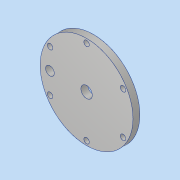
# Autodesk Inventor part: pistonSealingDisc
Saved by Autodesk Inventor 2017 (Build 210142000, 142)
## iProperties
Created: 2016-11-26
Part Number: pistonSealingDisc
Material: Aluminum 6061
Document SubType Name: Modeling
Designer: techn
Density: 2.7 g/cm^3
Appearance: Aluminum - Flat
Mass: 27.687 g
Surface Area: 74.4581 cm^2
Volume: 10.2545 cm^3
Author: techn
Autodesk Inventor part; units mm, degrees
ref_plane "YZ Plane" through (0, 0, 0) normal (1, 0, 0) x (0, 1, 0)
ref_plane "XZ Plane" through (0, 0, 0) normal (0, 1, 0) x (-1, 0, 0)
ref_plane "XY Plane" through (0, 0, 0) normal (0, 0, 1) x (1, 0, 0)
sketch "Sketch1" plane through (0, 0, 0) normal (0, 0, 1) x (1, 0, 0)
  circle A0 centre (0, 0) radius 32.1945
  dimension "d0" = 64.389
  constraints: 1 centre point, 1 coincident
  measures "d0" diameter of A0
extrude "Extrusion1" add sketch "Sketch1" along normal blind 4.7625
sketch "Sketch2" plane through (0, 0, 4.7625) normal (0, 0, 1) x (1, 0, 0)
  line L0 (0, 0) -> (0, 29.21)
  circle A0 centre (0, 29.21) radius 1.905
  circle A1 centre (-25.2966, 14.605) radius 1.905
  circle A2 centre (-25.2966, -14.605) radius 1.905
  circle A3 centre (0, -29.21) radius 1.905
  circle A4 centre (25.2966, -14.605) radius 1.905
  circle A5 centre (25.2966, 14.605) radius 1.905
  dimension "d3" = 29.21
  dimension "d4" = 3.81
  dimension "d7" = 360
  constraints: 6 centre point, 2 end point, 1 coincident, 1 vertical, 13 other
  measures "d3" distance of L0.start L0.end
  measures "d4" diameter of A0
extrude "Extrusion2" cut sketch "Sketch2" against normal through all
sketch "Sketch4" plane through (0, 0, 0) normal (0, 0, -1) x (-1, 0, 0)
  line L0 (0, 0) -> (25.4, 0)
  line L1 (20.0474, 0) -> (22.7237, 4.6355)
  line L2 (22.7237, 4.6355) -> (28.0763, 4.6355)
  line L3 (28.0763, 4.6355) -> (30.7526, 0)
  line L4 (30.7526, 0) -> (28.0763, -4.6355)
  line L5 (28.0763, -4.6355) -> (22.7237, -4.6355)
  line L6 (22.7237, -4.6355) -> (20.0474, 0)
  dimension "d12" = 25.4
  dimension "d13" = 9.271
  constraints: 14 end point, 1 coincident, 1 horizontal, 1 point on line, 13 other
  measures "d12" distance of L0.start L0.end
  measures "d13" distance between parallel lines of L5 L2
extrude "Extrusion3" cut sketch "Sketch4" against normal through all
sketch "Sketch5" plane through (0, 0, 0) normal (0, 0, -1) x (-1, 0, 0)
  line L0 (22.7237, -4.6355) -> (20.0474, 0) projected
  line L1 (20.0474, 0) -> (22.7237, 4.6355) projected
  line L2 (22.7237, 4.6355) -> (28.0763, 4.6355) projected
  line L3 (28.0763, 4.6355) -> (30.7526, 0) projected
  line L4 (30.7526, 0) -> (28.0763, -4.6355) projected
  line L5 (28.0763, -4.6355) -> (22.7237, -4.6355) projected
  circle A0 centre (0, 0) radius 32.1945 projected
  circle A1 centre (25.4, 0) radius 3.048
  line L6 (0, 0) -> (25.4, 0)
  dimension "d16" = 6.096
  dimension "d22" = 25.4
  constraints: 2 end point, 1 centre point, 1 horizontal
  measures "d16" diameter of A1
  measures "d22" distance of L6.start L6.end
extrude "Extrusion4" add sketch "Sketch5" against normal up to surface (4.7625 mm away) contours L0 L1 L2 L3 L4 L5
sketch "Sketch6" plane through (0, 0, 4.7625) normal (0, 0, 1) x (1, 0, 0)
  circle A0 centre (0, 0) radius 3.9624
  dimension "d19" = 7.9248
  constraints: 1 centre point, 1 coincident
  measures "d19" diameter of A0
extrude "Extrusion5" cut sketch "Sketch6" against normal through all
body "Solid1"
